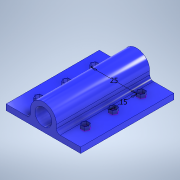
# Autodesk Inventor part: крепление направляющей руки
Saved by Autodesk Inventor 2020 (Build 240168000, 168)
## iProperties
Created: 2022-03-20
Part Number: крепление направляющей руки
Material: Типовые
Document SubType Name: Modeling
Designer: Администратор
Density: 1 g/cm^3
Appearance: По умолчанию
Author: Администратор
Autodesk Inventor part; units mm, degrees
ref_plane "YZ Plane" through (0, 0, 0) normal (1, 0, 0) x (0, 1, 0)
ref_plane "XZ Plane" through (0, 0, 0) normal (0, 1, 0) x (-1, 0, 0)
ref_plane "XY Plane" through (0, 0, 0) normal (0, 0, 1) x (1, 0, 0)
sketch "Эскиз1" plane through (0, 0, 0) normal (0, 0, 1) x (1, 0, 0)
  circle A0 centre (0, 0) radius 4.5
  line L0 (-9, -4) -> (-20, -4)
  line L1 (-20, -4) -> (-20, -5)
  line L2 (20, -5) -> (20, -4)
  line L3 (20, -4) -> (9, -4)
  line L4 (-20, -5) -> (-20, -7)
  line L5 (-20, -7) -> (20, -7)
  line L6 (20, -7) -> (20, -5)
  arc A1 (7, 0) -> (-7, 0) centre (0, 0) ccw
  line L7 (-7, 0) -> (-7, -2)
  line L8 (7, 0) -> (7, -2)
  arc A2 (-9, -4) -> (-7, -2) centre (-9, -2) ccw
  arc A3 (7, -2) -> (9, -4) centre (9, -2) ccw
  point P0 (3, -4)
  point P1 (-5, 0)
  point P2 (-5, -4)
  point P3 (5, 0)
  point P4 (5, -4)
  dimension "d0" = 9
  dimension "d2" = 1
  dimension "d20" = 2
  dimension "d21" = 14
  dimension "d22" = 2
  constraints: 18 end point, 6 point on circle, 5 perpendicular, 5 point on line, 5 tangent, 4 centre point, 2 coincident, 1 equal radius, 1 horizontal, 1 vertical
  measures "d0" diameter of A0
  measures "d2" distance of L0.end L1.end
  measures "d20" distance of L1.end L4.end
  measures "d21" diameter of A1
  measures "d22" radius of A2
extrude "Выдавливание4" add sketch "Эскиз1" along normal blind 50
sketch "Эскиз3" plane through (9, -4, 0) normal (0, 1, 0) x (1, 0, 0)
  circle A0 centre (-21.4987, -10) radius 1.5
  circle A1 centre (-21.4987, -25) radius 1.5
  circle A2 centre (-21.4987, -40) radius 1.5
  circle A3 centre (3.5013, -10) radius 1.5
  circle A4 centre (3.5013, -25) radius 1.5
  circle A5 centre (3.5013, -40) radius 1.5
  line L0 (5.2423, -9.8461) -> (4.5051, -11.4308)
  line L1 (4.5051, -11.4308) -> (2.7641, -11.5846)
  line L2 (2.7641, -11.5846) -> (1.7604, -10.1539)
  line L3 (1.7604, -10.1539) -> (2.4976, -8.5692)
  line L4 (2.4976, -8.5692) -> (4.2386, -8.4154)
  line L5 (4.2386, -8.4154) -> (5.2423, -9.8461)
  line L6 (2.3986, -8.2924) -> (4.4288, -8.1912)
  line L7 (4.4288, -8.1912) -> (5.5315, -9.8988)
  line L8 (5.5315, -9.8988) -> (4.604, -11.7076)
  line L9 (4.604, -11.7076) -> (2.5739, -11.8088)
  line L10 (2.5739, -11.8088) -> (1.4712, -10.1012)
  line L11 (1.4712, -10.1012) -> (2.3986, -8.2924)
  line L12 (3.5013, -10) -> (2.0013, -10)
  line L13 (3.5013, -10) -> (3.5013, -11.5)
  line L14 (1.4712, -25.1012) -> (2.3986, -23.2924)
  line L15 (2.3986, -23.2924) -> (4.4288, -23.1912)
  line L16 (4.4288, -23.1912) -> (5.5315, -24.8988)
  line L17 (4.2386, -23.4154) -> (5.2423, -24.8461)
  line L18 (2.4976, -23.5692) -> (4.2386, -23.4154)
  line L19 (1.7604, -25.1539) -> (2.4976, -23.5692)
  line L20 (2.7641, -26.5846) -> (1.7604, -25.1539)
  line L21 (2.5739, -26.8088) -> (1.4712, -25.1012)
  line L22 (4.604, -26.7076) -> (2.5739, -26.8088)
  line L23 (4.5051, -26.4308) -> (2.7641, -26.5846)
  line L24 (5.2423, -24.8461) -> (4.5051, -26.4308)
  line L25 (5.5315, -24.8988) -> (4.604, -26.7076)
  line L26 (1.4712, -40.1012) -> (2.3986, -38.2924)
  line L27 (2.3986, -38.2924) -> (4.4288, -38.1912)
  line L28 (4.4288, -38.1912) -> (5.5315, -39.8988)
  line L29 (4.2386, -38.4154) -> (5.2423, -39.8461)
  line L30 (2.4976, -38.5692) -> (4.2386, -38.4154)
  line L31 (1.7604, -40.1539) -> (2.4976, -38.5692)
  line L32 (2.7641, -41.5846) -> (1.7604, -40.1539)
  line L33 (2.5739, -41.8088) -> (1.4712, -40.1012)
  line L34 (4.604, -41.7076) -> (2.5739, -41.8088)
  line L35 (4.5051, -41.4308) -> (2.7641, -41.5846)
  line L36 (5.2423, -39.8461) -> (4.5051, -41.4308)
  line L37 (5.5315, -39.8988) -> (4.604, -41.7076)
  line L38 (-23.5288, -10.1012) -> (-22.6014, -8.2924)
  line L39 (-22.6014, -8.2924) -> (-20.5712, -8.1912)
  line L40 (-20.5712, -8.1912) -> (-19.4685, -9.8988)
  line L41 (-20.7614, -8.4154) -> (-19.7577, -9.8461)
  line L42 (-22.5024, -8.5692) -> (-20.7614, -8.4154)
  line L43 (-23.2396, -10.1539) -> (-22.5024, -8.5692)
  line L44 (-22.2359, -11.5846) -> (-23.2396, -10.1539)
  line L45 (-22.4261, -11.8088) -> (-23.5288, -10.1012)
  line L46 (-20.396, -11.7076) -> (-22.4261, -11.8088)
  line L47 (-20.4949, -11.4308) -> (-22.2359, -11.5846)
  line L48 (-19.7577, -9.8461) -> (-20.4949, -11.4308)
  line L49 (-19.4685, -9.8988) -> (-20.396, -11.7076)
  line L50 (-23.5288, -25.1012) -> (-22.6014, -23.2924)
  line L51 (-22.6014, -23.2924) -> (-20.5712, -23.1912)
  line L52 (-20.5712, -23.1912) -> (-19.4685, -24.8988)
  line L53 (-20.7614, -23.4154) -> (-19.7577, -24.8461)
  line L54 (-22.5024, -23.5692) -> (-20.7614, -23.4154)
  line L55 (-23.2396, -25.1539) -> (-22.5024, -23.5692)
  line L56 (-22.2359, -26.5846) -> (-23.2396, -25.1539)
  line L57 (-22.4261, -26.8088) -> (-23.5288, -25.1012)
  line L58 (-20.396, -26.7076) -> (-22.4261, -26.8088)
  line L59 (-20.4949, -26.4308) -> (-22.2359, -26.5846)
  line L60 (-19.7577, -24.8461) -> (-20.4949, -26.4308)
  line L61 (-19.4685, -24.8988) -> (-20.396, -26.7076)
  line L62 (-23.5288, -40.1012) -> (-22.6014, -38.2924)
  line L63 (-22.6014, -38.2924) -> (-20.5712, -38.1912)
  line L64 (-20.5712, -38.1912) -> (-19.4685, -39.8988)
  line L65 (-20.7614, -38.4154) -> (-19.7577, -39.8461)
  line L66 (-22.5024, -38.5692) -> (-20.7614, -38.4154)
  line L67 (-23.2396, -40.1539) -> (-22.5024, -38.5692)
  line L68 (-22.2359, -41.5846) -> (-23.2396, -40.1539)
  line L69 (-22.4261, -41.8088) -> (-23.5288, -40.1012)
  line L70 (-20.396, -41.7076) -> (-22.4261, -41.8088)
  line L71 (-20.4949, -41.4308) -> (-22.2359, -41.5846)
  line L72 (-19.7577, -39.8461) -> (-20.4949, -41.4308)
  line L73 (-19.4685, -39.8988) -> (-20.396, -41.7076)
  point P0 (-9, 0)
  dimension "d51" = 15
  dimension "d54" = 25
  constraints: 148 end point, 6 centre point, 2 horizontal, 2 point on circle, 2 vertical, 133 other
  measures "d51" distance of L10.end L14.start
  measures "d54" distance of L10.end L38.start
extrude "Выдавливание5" cut sketch "Эскиз3" against normal blind 3 contours A0
extrude "Выдавливание6" cut sketch "Эскиз3" against normal blind 3 contours A1 | A2 | A3 L13 L12 | L12 L13 A3 | A4 | A5
extrude "Выдавливание7" add sketch "Эскиз3" along normal blind 2 contours L6 L7 L8 L9 L10 L11 | L14 L15 L16 L25 L22 L21 | L26 L27 L28 L37 L34 L33 | L38 L39 L40 L49 L46 L45 | L50 L51 L52 L61 L58 L57 | L62 L63 L64 L73 L70 L69
